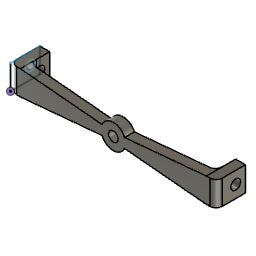
agarre de tuerca v2 brazo elevador (Autodesk Fusion 360 design; units mm, degrees)
Autodesk Fusion 360 part; units mm, degrees
sketch "Sketch1" plane through (0, 0, 0) normal (1, 0, 0) x (0, 1, 0)
  line L0 (0, 0) -> (12, 0)
  line L1 (12, 0) -> (12, 10)
  line L2 (12, 10) -> (0, 10)
  line L3 (0, 10) -> (0, 0)
  circle A0 centre (8, 5) radius 2
  dimension "d3" = 12
  dimension "d4" = 4
  constraint horizontal L0
  constraint vertical L1
  constraint horizontal L2
  constraint vertical L3
  constraint coincident L0.start L3.end
  measures "d3" distance of L1 L3
  measures "d4" diameter of A0
extrude "Extrude1" add sketch "Sketch1" along normal blind 4 contours L0 L1 L2 L3 | A0 makes body 1
extrude "Extrude2" add sketch "Sketch1" along normal blind 4 separate body makes body 2
extrude "Extrude4" cut sketch "Sketch1" along normal blind 125 contours A0 bodies 1
sketch "Sketch3" plane through (0, 6, 5) normal (1, 0, 0) x (0, 1, 0)
  line L0 (-6, 5) -> (-2, 5)
  line L1 (-2, 5) -> (-2, -5)
  line L2 (-6, -5) -> (-6, 5)
  line L3 (-2, -5) -> (-6, -5)
  constraint horizontal L0
  constraint perpendicular L0 L1
  constraint perpendicular L0 L2
  constraint perpendicular L2 L3
extrude "Extrude5" add sketch "Sketch3" along normal blind 80 bodies 1 2
sketch "Sketch4" plane through (0, 4, 0) normal (0, 1, 0) x (-1, 0, 0)
  line L0 (-4, 0) -> (-4, 10)
  line L1 (-4, 10) -> (-80, 10)
  line L2 (-80, 10) -> (-80, 0)
  line L3 (-80, 0) -> (-4, 0)
  circle A0 centre (-42, 5) radius 2
extrude "Extrude6" cut sketch "Sketch4" against normal blind 14 contours A0 bodies 1
sketch "Sketch5" plane through (0, 0, 10) normal (0, 0, 1) x (-1, 0, 0)
  line L0 (-4, -4) -> (-4, -12)
  line L1 (-4, -12) -> (0, -12)
  line L2 (0, -12) -> (0, 0)
  line L3 (0, 0) -> (-80, 0)
  line L4 (-80, 0) -> (-80, -4)
  line L5 (-80, -4) -> (-4, -4)
  line L6 (-80, 0) -> (-84, 0)
  line L7 (-84, 0) -> (-84, -12)
  line L8 (-84, -12) -> (-80, -12)
  line L9 (-80, -12) -> (-80, 0)
  dimension "d15" = 4
  constraint coincident L3.end L4.start
  constraint perpendicular L4 L6
  constraint perpendicular L1 L7
  constraint perpendicular L7 L8
  constraint parallel L4 L9
  measures "d15" distance of L3.end L6.end
extrude "Extrude7" add sketch "Sketch5" against normal blind 10 contours L4 L6 L7 L8 L9 bodies 1
extrude "Extrude8" cut sketch "Sketch1" along normal blind 360 contours A0 bodies 1
sketch "Sketch6" plane through (0, 4, 0) normal (0, 1, 0) x (-1, 0, 0)
  circle A0 centre (-42, 5) radius 2
  line L0 (-4, 0) -> (-4, 10)
  line L1 (-4, 10) -> (-80, 10)
  line L2 (-80, 10) -> (-80, 0)
  line L3 (-80, 0) -> (-4, 0)
  circle A1 centre (-42, 5) radius 5
  line L4 (-42, 5) -> (-40, 5)
  line L5 (-37, 5) -> (-47, 5)
  line L6 (-37, 5) -> (-37.5116, 6.9335)
  line L7 (-47, 5) -> (-46.4882, 6.9334)
  line L8 (-47, 5) -> (-46.6078, 3.0388)
  line L9 (-37, 5) -> (-37.5177, 3.0682)
  line L10 (-46.4882, 6.9334) -> (-80, 10)
  line L11 (-46.6078, 3.0388) -> (-80, 0)
  line L12 (-37.5116, 6.9335) -> (-4, 10)
  line L13 (-37.5177, 3.0682) -> (-4, 0)
  dimension "d20" = 2
  dimension "d21" = 2
  dimension "d22" = 2
  dimension "d23" = 2
  constraint concentric A0 A1
  constraint tangent L1 A1
  constraint coincident A0.centre A1.centre
  constraint coincident A0 L4.end
  constraint horizontal L4
  constraint coincident A1 L5.start
  constraint coincident A1 L5.end
  constraint parallel L4 L5
  constraint coincident L1.end L2.start
  constraint coincident L2.end L3.start
  constraint coincident L0.end L1.start
  constraint coincident L0.start L3.end
  measures "d20" distance of L5.start L6.end
  measures "d21" distance of L5.end L7.end
  measures "d22" distance of L5.end L8.end
  measures "d23" distance of L5.start L9.end
extrude "Extrude9" cut sketch "Sketch6" against normal blind 20 contours L1 A1 L12 | L3 A1 L13 | L1 A1 L10 | L3 A1 L8 L11 bodies 1
fillet "Fillet1" radius 2.5 4 edges at (0, 0, 5) (84, 0, 5) (80, 4, 5) (4, 4, 5) on bodies 1
